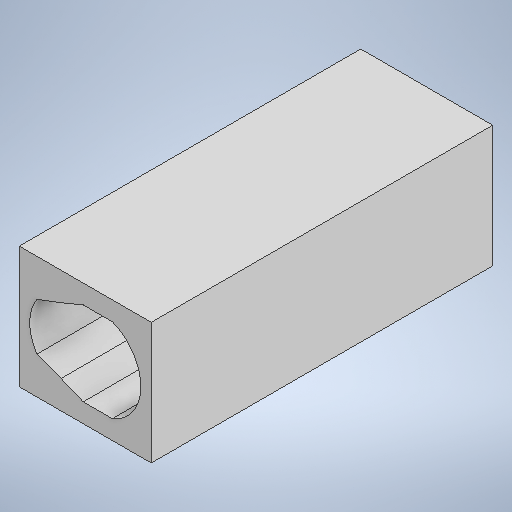
# Autodesk Inventor part: SLEEVE
Saved by Autodesk Inventor 2025.1 (Build 291241000, 241)
## iProperties
Created: 2025-01-31
Part Number: SLEEVE
Material: Generic
Document SubType Name: Modeling
Designer: 13156
Density: 1 g/cm^3
Appearance: Default
Author: 13156
Autodesk Inventor part; units mm, degrees
ref_plane "YZ Plane" through (0, 0, 0) normal (1, 0, 0) x (0, 1, 0)
ref_plane "XZ Plane" through (0, 0, 0) normal (0, 1, 0) x (-1, 0, 0)
ref_plane "XY Plane" through (0, 0, 0) normal (0, 0, 1) x (1, 0, 0)
sketch "Sketch1" plane through (0, 0, 0) normal (0, 0, 1) x (1, 0, 0)
  line L0 (-19.5, 18) -> (19.5, 18)
  line L1 (19.5, 18) -> (19.5, -18)
  line L2 (19.5, -18) -> (-19.5, -18)
  line L3 (-19.5, -18) -> (-19.5, 18)
  line L4 (-10.1739, 0) -> (5.8261, 0) construction
  line L5 (0, 4.6624) -> (0, -4.6624) construction
  point P0 (0, 0)
  point P1 (0, 0)
  point P2 (19.5, 0)
  dimension "d1" = 36
  dimension "d2" = 39
  dimension "d4" = 0
  dimension "d5" = 18
  dimension "d6" = 19.5
  constraints: 12 end point, 2 horizontal, 2 midpoint, 2 parallel, 1 perpendicular, 1 vertical, 2 other
  measures "d1" distance of L0.end L1.end
  measures "d2" distance of L0.start L0.end
  measures "d4" distance from line of point (0, 0) L5
  measures "d5" distance from line of L2 point (0, 0)
  measures "d6" distance of point (19.5, 0) point (0, 0)
extrude "Extrusion1" add sketch "Sketch1" along normal blind 100.9
sketch "Sketch2" plane through (0, 0, 100.9) normal (0, 0, 1) x (1, 0, 0)
  arc A0 (8.0072, -12.4) -> (8.0072, 12.4) centre (3.0434, 0) ccw
  line L0 (8.0072, 12.4) -> (-0.5928, 12.4)
  line L1 (8.0072, -12.4) -> (-0.5928, -12.4)
  line L2 (-0.5928, 12.4) -> (-7.1493, 9.7)
  line L3 (-0.5928, -12.4) -> (-7.1493, -9.7)
  line L4 (-7.1493, 9.7) -> (-14.2493, 7)
  line L5 (-7.1493, -9.7) -> (-14.2493, -7)
  arc A1 (-14.2493, 7) -> (-14.2493, -7) centre (-3.9328, 0) ccw
  line L6 (8.0072, -12.4) -> (8.0072, 12.4) construction
  line L7 (-18.7661, 0) -> (23.2506, 0) construction
  line L8 (-0.5928, -12.4) -> (-0.5928, 12.4) construction
  line L9 (-14.2493, -7) -> (-14.2493, 7.95) construction
  line L10 (-0.3392, 0) -> (0.4875, 0) construction
  line L11 (-19.5, -18) -> (19.5, -18) projected
  line L12 (19.5, 18) -> (-19.5, 18) projected
  line L13 (19.5, -18) -> (19.5, 18) projected
  point P0 (-0.9278, -0.8319)
  point P1 (16.4, 0)
  point P2 (-16.4, 0)
  point P3 (3.7072, -12.4)
  point P4 (-18.969, 0)
  point P5 (2.2423, 0)
  point P6 (0.0742, 0)
  dimension "d11" = 32.8
  dimension "d12" = 24.8
  dimension "d13" = 14
  dimension "d14" = 7.1
  dimension "d15" = 6.5566
  dimension "d16" = 2.7
  dimension "d17" = 13.3566
  dimension "d18" = 12.4672
  dimension "d19" = 2.569
  dimension "d20" = 24.8
  dimension "d21" = 3.1701
  dimension "d22" = 0.8319
  dimension "d23" = 0.335
  dimension "d26" = 0
  dimension "d28" = 5.6
  dimension "d29" = 3.1
  constraints: 22 end point, 6 point on circle, 4 horizontal, 3 equal length, 3 midpoint, 2 centre point, 1 point on line, 1 vertical, 3 other
  measures "d11" distance of point (-16.4, 0) point (16.4, 0)
  measures "d12" distance from line of L0 point (3.707, -12.4)
  measures "d13" distance of L4.end L5.end
  measures "d14" horizontal distance of L3.end L5.end
  measures "d15" horizontal distance of L1.end L3.end
  measures "d16" vertical distance of L1.end L3.end
  measures "d17" radius of A0
  measures "d18" radius of A1
  measures "d19" distance of point (-18.969, 0) point (-16.4, 0)
  measures "d20" distance of L6.end L1.start
  measures "d21" horizontal distance of point (-0.928, -0.832) point (2.242, 0)
  measures "d22" vertical distance of point (-0.928, -0.832) point (2.242, 0)
  measures "d23" distance from line of point (-0.928, -0.832) L8
  measures "d26" distance from line of L7 point (0.074, 0)
  measures "d28" distance between parallel lines of L12 L0
  measures "d29" distance from line of L13 point (16.4, 0)
extrude "Extrusion2" cut sketch "Sketch2" against normal blind 100.9 draft -0.2
sketch "Sketch3" plane through (0, 0, 0) normal (0, 0, -1) x (-1, 0, 0)
  line L0 (13.561, -5.8151) -> (0.5231, -10.7732)
  line L1 (7.1493, -9.7) -> (14.2493, -7) projected
  arc A0 (13.561, -5.8151) -> (13.561, 5.8151) centre (2.9328, 0) ccw
  arc A1 (14.0195, -6.7106) -> (14.0195, 6.7106) centre (3.9328, 0) ccw projected
  line L2 (14.0195, -6.7106) -> (7.0197, -9.3725) projected
  line L3 (0.5231, -12.0478) -> (-7.9389, -12.0478) projected
  line L4 (0.5231, -12.0478) -> (0.5231, 13.0926) construction
  arc A2 (14.2493, -7) -> (14.2493, 7) centre (3.9328, 0) ccw construction
  line L5 (16.4, 0) -> (-18.8741, 0) construction
  line L6 (13.561, 5.8151) -> (0.5231, 10.7732)
  arc A3 (-7.9389, 12.0478) -> (-7.9389, -12.0478) centre (-3.0434, 0) ccw projected
  line L7 (-7.9389, 12.0478) -> (0.5231, 12.0478) projected
  line L8 (-7.9389, -12.0478) -> (-7.9389, 12.0478) construction
  line L9 (19.5, 18) -> (19.5, -18) projected
  line L10 (19.5, -18) -> (-19.5, -18)
  line L11 (-19.5, -18) -> (-19.5, 18)
  line L12 (-19.5, 18) -> (19.5, 18)
  line L13 (19.5, 18) -> (19.5, -18)
  line L14 (0.5231, 10.7732) -> (-7.9389, 10.7732)
  line L15 (19.5, 0) -> (-18.8741, 0) construction
  line L16 (0.5231, -10.7732) -> (-7.9389, -10.7732)
  arc A4 (-7.9389, 10.7732) -> (-7.9389, -10.7732) centre (-3.3303, 0) ccw
  point P0 (0, 0)
  point P1 (-16.0478, 0)
  point P2 (16.0478, 0)
  point P3 (15.0478, 0)
  point P4 (-16.0478, 0)
  point P5 (-16.0478, 0)
  point P6 (-15.0478, 0)
  dimension "d33" = 1
  dimension "d39" = 1
  dimension "d42" = 0
  dimension "d47" = 0
  dimension "d48" = 1
  dimension "d49" = 0.8955
  constraints: 24 end point, 11 point on circle, 3 horizontal, 3 parallel, 3 perpendicular, 2 centre point, 2 point on line, 2 vertical, 1 equal radius, 1 midpoint, 1 other
  measures "d33" distance between parallel lines of L0 L2
  measures "d39" distance of point (16.048, 0) point (15.048, 0)
  measures "d42" distance from line of L4 L0.end
  measures "d47" distance from line of L4 L6.end
  measures "d48" distance of point (-16.048, 0) point (-15.048, 0)
  measures "d49" vertical distance of A1.end L6.start
extrude "Extrusion3" add sketch "Sketch3" against normal blind 2
body "Solid1"
